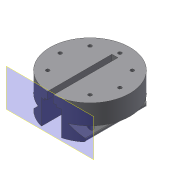
# Autodesk Inventor part: arm_0_attachment
Saved by Autodesk Inventor 2018 (Build 220112000, 112)
## iProperties
Created: 2017-12-03
Part Number: arm_0_attachment
Material: Generic
Document SubType Name: Modeling
Designer: Bardo91
Density: 1 g/cm^3
Appearance: Default
Author: Bardo91
Autodesk Inventor part; units mm, degrees
ref_plane "YZ Plane" through (0, 0, 0) normal (1, 0, 0) x (0, 1, 0)
ref_plane "XY Plane" through (0, 0, 0) normal (0, 0, 1) x (1, 0, 0)
sketch "Sketch1" plane through (0, 0, 0) normal (0, 0, 1) x (1, 0, 0)
  circle A0 centre (0, 0) radius 40
  dimension "d0" = 80
  constraints: 1 centre point, 1 coincident
  measures "d0" diameter of A0
extrude "base" add sketch "Sketch1" along normal blind 20
sketch "Sketch2" plane through (0, 0, 0) normal (0, 1, 0) x (-1, 0, 0)
  line L0 (0, 0) -> (15, 0)
  line L1 (-40, 0) -> (40, 0) projected
  line L2 (15, 0) -> (29.1421, -14.1421)
  line L3 (0, 0) -> (-15, 0)
  line L4 (-15, 0) -> (-29.1421, -14.1421)
  line L5 (-29.1421, -14.1421) -> (29.1421, -14.1421)
  dimension "d3" = 15
  dimension "d4" = 20
  dimension "d5" = 135
  dimension "d6" = 15
  dimension "d7" = 20
  dimension "d8" = 135
  constraints: 10 end point, 2 point on line
  measures "d3" distance of L0.start L0.end
  measures "d4" distance of L0.end L2.end
  measures "d5" angle of L0 L2
  measures "d6" distance of L0.start L3.end
  measures "d7" distance of L3.end L4.end
  measures "d8" angle of L4 L3
extrude "tail_horse_1" add sketch "Sketch2" along normal up to surface round surface about axis through (0, 0, 0) along (0, 0, 1) radius 40 far side no
mirror "tail_horse_2" about plane through (0, 0, -8.6301) normal (0, -1, 0) of "tail_horse_1"
fillet "fillet_tail_horse" radius 2 2 edges at (-29.1421, 0, -14.1421) (29.1421, 0, -14.1421)
sketch "Sketch3" plane through (0, 0, 20) normal (0, 0, 1) x (1, 0, 0)
  line L0 (0, 0) -> (0, -30)
  circle A0 centre (0, -30) radius 1.75
  circle A1 centre (21.2132, -21.2132) radius 1.75
  circle A2 centre (30, 0) radius 1.75
  circle A3 centre (21.2132, 21.2132) radius 1.75
  circle A4 centre (0, 30) radius 1.75
  circle A5 centre (-21.2132, 21.2132) radius 1.75
  circle A6 centre (-30, 0) radius 1.75
  circle A7 centre (-21.2132, -21.2132) radius 1.75
  dimension "d12" = 30
  dimension "d13" = 3.5
  dimension "d16" = 360
  constraints: 8 centre point, 2 end point, 1 coincident, 1 vertical, 17 other
  measures "d12" distance of L0.start L0.end
  measures "d13" diameter of A0
extrude "attach_screw" cut sketch "Sketch3" against normal through all
sketch "Sketch4" plane through (0, 0, -14.1421) normal (0, 0, -1) x (-1, 0, 0)
  line L0 (0, 0) -> (0, 30)
  circle A0 centre (0, 30) radius 3
  circle A1 centre (-21.2132, 21.2132) radius 3
  circle A2 centre (-30, 0) radius 3
  circle A3 centre (-21.2132, -21.2132) radius 3
  circle A4 centre (0, -30) radius 3
  circle A5 centre (21.2132, -21.2132) radius 3
  circle A6 centre (30, 0) radius 3
  circle A7 centre (21.2132, 21.2132) radius 3
  dimension "d20" = 30
  dimension "d21" = 6
  dimension "d24" = 360
  constraints: 8 centre point, 2 end point, 1 coincident, 1 vertical, 17 other
  measures "d20" distance of L0.start L0.end
  measures "d21" diameter of A0
extrude "attach_screw_head" cut sketch "Sketch4" against normal blind 20
sketch "Sketch5" plane through (0, 0, 0) normal (1, 0, 0) x (0, 1, 0)
  line L0 (31.7623, -14.1421) -> (-31.7623, -14.1421) projected
  line L1 (0, -14.1421) -> (0, -6.1421)
  circle A0 centre (0, -6.1421) radius 1.75
  point P0 (0, 0)
  dimension "d28" = 8
  dimension "d29" = 3.5
  constraints: 2 end point, 1 centre point, 1 coincident, 1 midpoint, 1 vertical
  measures "d28" distance of L1.start L1.end
  measures "d29" diameter of A0
extrude "lock_arm" cut sketch "Sketch5" along normal through all both and the other way through all
ref_plane "Work Plane1" through (0, -40, 0) normal (0, 1, 0) x (-1, 0, 0)
sketch "Sketch6" plane through (0, -40, 0) normal (0, 1, 0) x (-1, 0, 0)
  line L0 (24.3137, -14.1421) -> (-24.3137, -14.1421) projected
  line L1 (0, -14.1421) -> (10, -14.1421)
  line L2 (10, -14.1421) -> (10, 10.8579)
  line L3 (10, 10.8579) -> (-10, 10.8579)
  line L4 (-10, 10.8579) -> (-10, -14.1421)
  line L5 (0, -14.1421) -> (-10, -14.1421)
  line L6 (0, 10.8579) -> (6, 10.8579)
  line L7 (6, 10.8579) -> (6, 12.8579)
  line L8 (6, 12.8579) -> (3, 12.8579)
  line L9 (3, 12.8579) -> (3, 20)
  line L10 (0, 10.8579) -> (-6, 10.8579)
  line L11 (-6, 10.8579) -> (-6, 12.8579)
  line L12 (-6, 12.8579) -> (-3, 12.8579)
  line L13 (-3, 12.8579) -> (-3, 20)
  line L14 (-3, 20) -> (3, 20)
  point P0 (0, 0)
  dimension "d32" = 10
  dimension "d33" = 25
  dimension "d34" = 20
  dimension "d37" = 6
  dimension "d38" = 2
  dimension "d39" = 3
  dimension "d40" = 6
  dimension "d41" = 3
  constraints: 28 end point, 10 perpendicular, 4 point on line, 2 midpoint, 1 vertical
  measures "d32" distance of L1.start L1.end
  measures "d33" distance of L1.end L2.end
  measures "d34" distance of L2.end L3.end
  measures "d37" distance of L6.start L6.end
  measures "d38" distance of L6.end L7.end
  measures "d39" distance of L7.end L8.end
  measures "d40" distance of L6.start L10.end
  measures "d41" distance of L11.end L12.end
extrude "servo_place" cut sketch "Sketch6" along normal blind 65
equation "\"d6\" = d3"
equation "\"d7\" = d4"
equation "\"d8\" = d5"
body "Solid1"
